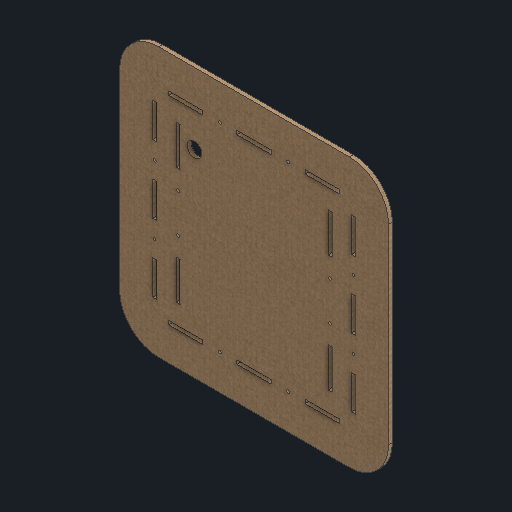
# Autodesk Inventor part: Cover
Saved by Autodesk Inventor 2024.1 (Build 281209000, 209)
## iProperties
Created: 2023-08-05
Part Number: Cover
Material: MDF Medium Density Fiberboard
Document SubType Name: Modeling
Designer: jaege
Density: 0.8 g/cm^3
Appearance: Cardboard - Corrugated
Author: jaege
Autodesk Inventor part; units mm, degrees
ref_plane "YZ Plane" through (0, 0, 0) normal (1, 0, 0) x (0, 1, 0)
ref_plane "XZ Plane" through (0, 0, 0) normal (0, 1, 0) x (-1, 0, 0)
ref_plane "XY Plane" through (0, 0, 0) normal (0, 0, 1) x (1, 0, 0)
sketch "Sketch1" plane through (0, 0, 0) normal (0, 0, 1) x (1, 0, 0)
  line L0 (6, 225.5) -> (202, 225.5)
  line L1 (242, 185.5) -> (242, -10.5)
  line L2 (202, -50.5) -> (6, -50.5)
  line L3 (-34, -10.5) -> (-34, 185.5)
  line L4 (208, 237.5) -> (0, 237.5) construction
  line L5 (-46, 191.5) -> (-46, -16.5) construction
  arc A0 (0, 237.5) -> (-46, 191.5) centre (0, 191.5) ccw construction
  arc A1 (6, 225.5) -> (-34, 185.5) centre (6, 185.5) ccw
  arc A2 (242, 185.5) -> (202, 225.5) centre (202, 185.5) ccw
  arc A3 (202, -50.5) -> (242, -10.5) centre (202, -10.5) ccw
  arc A4 (-34, -10.5) -> (6, -50.5) centre (6, -10.5) ccw
  line L6 (51.5, 191.5) -> (16.5, 191.5) projected
  line L7 (16.5, 191.5) -> (16.5, 187.5) projected
  line L8 (51.5, 187.5) -> (16.5, 187.5) projected
  line L9 (51.5, 191.5) -> (51.5, 187.5) projected
  line L10 (121.5, 191.5) -> (86.5, 191.5) projected
  line L11 (86.5, 191.5) -> (86.5, 187.5) projected
  line L12 (121.5, 187.5) -> (86.5, 187.5) projected
  line L13 (121.5, 191.5) -> (121.5, 187.5) projected
  line L14 (191.5, 191.5) -> (156.5, 191.5) projected
  line L15 (156.5, 191.5) -> (156.5, 187.5) projected
  line L16 (191.5, 187.5) -> (156.5, 187.5) projected
  line L17 (191.5, 191.5) -> (191.5, 187.5) projected
  line L18 (208, 140) -> (208, 175) projected
  line L19 (208, 175) -> (204, 175) projected
  line L20 (204, 140) -> (204, 175) projected
  line L21 (208, 140) -> (204, 140) projected
  line L22 (208, 70) -> (208, 105) projected
  line L23 (208, 105) -> (204, 105) projected
  line L24 (204, 70) -> (204, 105) projected
  line L25 (208, 70) -> (204, 70) projected
  line L26 (208, 0) -> (208, 35) projected
  line L27 (208, 35) -> (204, 35) projected
  line L28 (204, 0) -> (204, 35) projected
  line L29 (208, 0) -> (204, 0) projected
  line L30 (156.5, -16.5) -> (191.5, -16.5) projected
  line L31 (191.5, -16.5) -> (191.5, -12.5) projected
  line L32 (156.5, -12.5) -> (191.5, -12.5) projected
  line L33 (156.5, -16.5) -> (156.5, -12.5) projected
  line L34 (86.5, -16.5) -> (121.5, -16.5) projected
  line L35 (121.5, -16.5) -> (121.5, -12.5) projected
  line L36 (86.5, -12.5) -> (121.5, -12.5) projected
  line L37 (86.5, -16.5) -> (86.5, -12.5) projected
  line L38 (16.5, -16.5) -> (51.5, -16.5) projected
  line L39 (51.5, -16.5) -> (51.5, -12.5) projected
  line L40 (16.5, -12.5) -> (51.5, -12.5) projected
  line L41 (16.5, -16.5) -> (16.5, -12.5) projected
  line L42 (0, 35) -> (0, 0) projected
  line L43 (0, 0) -> (4, 0) projected
  line L44 (4, 35) -> (4, 0) projected
  line L45 (0, 35) -> (4, 35) projected
  line L46 (0, 105) -> (0, 70) projected
  line L47 (0, 70) -> (4, 70) projected
  line L48 (4, 105) -> (4, 70) projected
  line L49 (0, 105) -> (4, 105) projected
  line L50 (0, 175) -> (0, 140) projected
  line L51 (0, 140) -> (4, 140) projected
  line L52 (4, 175) -> (4, 140) projected
  line L53 (0, 175) -> (4, 175) projected
  circle A5 centre (43, 152.5) radius 7.5
  line L54 (4, 180) -> (4, 165) projected
  line L55 (24, 7.5) -> (28, 7.5)
  line L56 (28, 7.5) -> (28, 47.5)
  line L57 (28, 47.5) -> (24, 47.5)
  line L58 (24, 47.5) -> (24, 7.5)
  line L59 (180, 7.5) -> (184, 7.5)
  line L60 (184, 7.5) -> (184, 47.5)
  line L61 (184, 47.5) -> (180, 47.5)
  line L62 (180, 47.5) -> (180, 7.5)
  line L63 (180, 127.5) -> (184, 127.5)
  line L64 (184, 127.5) -> (184, 167.5)
  line L65 (184, 167.5) -> (180, 167.5)
  line L66 (180, 167.5) -> (180, 127.5)
  line L67 (24, 127.5) -> (28, 127.5)
  line L68 (28, 127.5) -> (28, 167.5)
  line L69 (28, 167.5) -> (24, 167.5)
  line L70 (24, 167.5) -> (24, 127.5)
  line L71 (104, 187.5) -> (104, -12.5) construction
  circle A6 centre (26, 107.5) radius 1.5
  circle A7 centre (26, 67.5) radius 1.5
  circle A8 centre (182, 107.5) radius 1.5
  circle A9 centre (182, 67.5) radius 1.5
  line L72 (26, 127.5) -> (26, 107.5) construction
  line L73 (26, 67.5) -> (26, 47.5) construction
  line L74 (26, 107.5) -> (26, 87.5) construction
  line L75 (26, 87.5) -> (26, 67.5) construction
  line L76 (51.5, 191.5) -> (86.5, 187.5) construction
  line L77 (121.5, 187.5) -> (156.5, 191.5) construction
  circle A10 centre (69, 189.5) radius 1.5
  circle A11 centre (139, 189.5) radius 1.5
  circle A12 centre (2, 122.5) radius 1.5
  circle A13 centre (2, 52.5) radius 1.5
  circle A14 centre (69, -14.5) radius 1.5
  circle A15 centre (139, -14.5) radius 1.5
  circle A16 centre (206, 52.5) radius 1.5
  circle A17 centre (206, 122.5) radius 1.5
  point P0 (104, 237.5)
  point P1 (104, 225.5)
  point P2 (-34, 87.5)
  point P3 (-46, 87.5)
  point P4 (-24, 191.5)
  point P5 (4, 172.5)
  point P6 (182, 127.5)
  point P7 (182, 47.5)
  point P8 (104, 87.5)
  dimension "d0" = 10
  dimension "d2" = 40
  dimension "d4" = 15
  dimension "d6" = 4
  dimension "d7" = 40
  dimension "d9" = 20
  dimension "d10" = 4
  dimension "d11" = 40
  dimension "d12" = 4
  dimension "d13" = 40
  dimension "d14" = 4
  dimension "d15" = 40
  dimension "d16" = 20
  dimension "d17" = 15
  dimension "d18" = 15
  dimension "d19" = 20
  dimension "d22" = 3
  dimension "d24" = 3
  dimension "d27" = 360
  constraints: 54 end point, 17 centre point, 15 equal length, 14 midpoint, 8 point on circle, 8 tangent, 7 equal radius, 5 horizontal, 5 perpendicular, 5 vertical alignment, 3 horizontal alignment, 2 symmetric about line, 2 vertical, 19 other
  measures "d0" distance from line of L3 point (-24, 191.5)
  measures "d2" radius of A1
  measures "d4" diameter of A5
  measures "d6" distance of L57.end L56.end
  measures "d7" distance of L56.end L55.end
  measures "d9" distance from line of L40 L55.end
  measures "d10" distance of L61.end L61.start
  measures "d11" distance of L61.start L59.end
  measures "d12" distance of L65.end L65.start
  measures "d13" distance of L65.start L63.end
  measures "d14" distance of L69.end L69.start
  measures "d15" distance of L69.start L67.end
  measures "d16" distance from line of L16 L65.start
  measures "d17" horizontal distance of A5.centre L69.start
  measures "d18" distance from line of A5.centre L68
  measures "d19" distance between parallel lines of L44 L58
  measures "d22" diameter of A6
  measures "d24" diameter of A10
extrude "Extrusion1" add sketch "Sketch1" along normal blind 4
body "Solid1"
